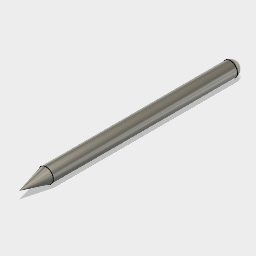
TEST2 (Autodesk Fusion 360 design; units mm, degrees)
Autodesk Fusion 360 part; units mm, degrees
cylinder "圆柱体基本要素1" add diameter 8 height 100 placed x (1, 0, 0) y (0, 0, -1) z (0, 1, 0) at (0, 0, 0) makes body 1
move_body "移动1" bodies 1 to x (1, 0, 0) y (0, 0, -1) z (0, 1, 0) at (-64.3143, -62.3311, -4)
sphere "球体基本要素1" add diameter 8 placed x (1, 0, 0) y (0, 0, -1) z (0, 1, 0) at (-57.404, 0, -63.1423) separate body makes body 2
move_body "对齐1" bodies 2 to x (1, 0, 0) y (0, 1, 0) z (0, 0, 1) at (-6.9103, -62.3311, -40.8577)
sketch "草图3" plane through (0, 0, 0) normal (0, 1, 0) x (1, 0, 0)
  line L0 (-30.3364, 31.7893) -> (-30.3364, 16.7893)
  line L1 (-30.3364, 16.7893) -> (-26.3364, 16.7893)
  line L2 (-30.3364, 31.7893) -> (-26.3364, 16.7893)
  dimension "d4" = 15
  dimension "d5" = 4
  measures "d4" distance of L0.start L0.end
  measures "d5" distance of L0.end L1.end
revolve "旋转1" add sketch "草图3" angle 360 about axis through (-30.3364, 0, -31.7893) along (0, 0, 1) separate body makes body 3
move_body "对齐2" bodies 3 to x (-1, 0, 0) y (0, 1, 0) z (0, 0, -1) at (-94.6508, -62.3311, -20.7893)
combine "合并1" operation add target body 1 tool bodies 2 3
